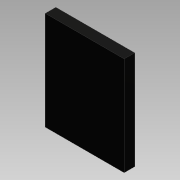
# Autodesk Inventor part: Ak-C-C39-USB-board
Saved by Autodesk Inventor 2016 (Build 200138000, 138)
## iProperties
Created: 2016-06-09
Part Number: Ak-C-C39-USB-board
Material: Generic
Document SubType Name: Modeling
Designer: admin
Density: 1 g/cm^3
Appearance: Default
Mass: 0.288 g
Surface Area: 4.464 cm^2
Volume: 0.288 cm^3
Author: admin
Autodesk Inventor part; units mm, degrees
ref_plane "YZ Plane" through (0, 0, 0) normal (1, 0, 0) x (0, 1, 0)
ref_plane "XZ Plane" through (0, 0, 0) normal (0, 1, 0) x (-1, 0, 0)
ref_plane "XY Plane" through (0, 0, 0) normal (0, 0, 1) x (1, 0, 0)
sketch "Sketch1" plane through (0, 0, 0) normal (0, 1, 0) x (-1, 0, 0)
  line L0 (6, 7.5) -> (-6, 7.5)
  line L1 (-6, 7.5) -> (-6, -7.5)
  line L2 (-6, -7.5) -> (6, -7.5)
  line L3 (6, -7.5) -> (6, 7.5)
  point P0 (0, 0)
  point P1 (0, -7.5)
  point P2 (6, 0)
  dimension "d0" = 12
  dimension "d1" = 15
  constraints: 8 end point, 2 midpoint, 2 parallel, 1 horizontal, 1 horizontal alignment, 1 perpendicular, 1 vertical alignment
  measures "d0" distance between parallel lines of L1 L3
  measures "d1" distance between parallel lines of L0 L2
extrude "Extrusion1" add sketch "Sketch1" along normal blind 1.6
body "Solid1"
